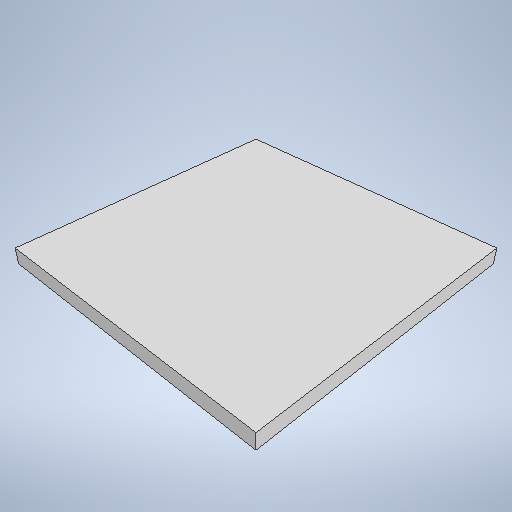
# Autodesk Inventor part: qr
Saved by Autodesk Inventor 2025.1 (Build 291241000, 241)
## iProperties
Created: 2024-10-19
Part Number: qr
Material: Generic
Document SubType Name: Modeling
Designer: VINCENT OGWENO
Density: 1 g/cm^3
Appearance: Default
Author: VINCENT OGWENO
Autodesk Inventor part; units mm, degrees
ref_plane "YZ Plane" through (0, 0, 0) normal (1, 0, 0) x (0, 1, 0)
ref_plane "XZ Plane" through (0, 0, 0) normal (0, 1, 0) x (-1, 0, 0)
ref_plane "XY Plane" through (0, 0, 0) normal (0, 0, 1) x (1, 0, 0)
sketch "Sketch1" plane through (0, 0, 0) normal (0, 1, 0) x (-1, 0, 0)
  line L0 (0, 0) -> (-350, 0)
  line L1 (-350, 0) -> (-350, 350)
  line L2 (-350, 350) -> (0, 350)
  line L3 (0, 350) -> (0, 0)
  dimension "d0" = 350
  dimension "d1" = 350
  constraints: 8 end point, 2 parallel, 1 horizontal, 1 perpendicular
  measures "d0" distance of L2.end L0.start
  measures "d1" distance from line of L3 L0.end
extrude "Extrusion1" add sketch "Sketch1" along normal blind 20
body "Solid1"
